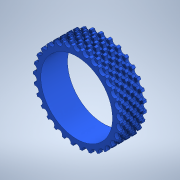
# Autodesk Inventor part: 3inBlueTread
Saved by Autodesk Inventor 2020 (Build 240168000, 168)
## iProperties
Created: 2019-05-28
Part Number: 3inBlueTread
Material: Generic
Document SubType Name: Modeling
Designer: Connor
Density: 1 g/cm^3
Appearance: Rubber - Blue
Author: Connor
Autodesk Inventor part; units mm, degrees
ref_plane "YZ Plane" through (0, 0, 0) normal (1, 0, 0) x (0, 1, 0)
ref_plane "XZ Plane" through (0, 0, 0) normal (0, 1, 0) x (-1, 0, 0)
ref_plane "XY Plane" through (0, 0, 0) normal (0, 0, 1) x (1, 0, 0)
sketch "Sketch1" plane through (0, 0, 0) normal (0, 0, 1) x (1, 0, 0)
  circle A0 centre (0, 0) radius 41.2242
  circle A1 centre (0, 0) radius 34.1122
  dimension "d3" = 7.112
  dimension "d4" = 68.2244
  constraints: 2 centre point, 1 coincident
  measures "d3" radial gap between concentric circles of A0 A1
  measures "d4" diameter of A1
extrude "Extrusion1" add sketch "Sketch1" along normal blind 25.4
sketch "Sketch3" plane through (0, 0, 25.4) normal (0, 0, 1) x (1, 0, 0)
  circle A0 centre (0, 0) radius 41.2242 projected
  arc A1 (-3.1726, 41.1019) -> (3.1726, 41.1019) centre (0, 41.2242) ccw
  circle A2 centre (0, 0) radius 41.2242 projected
  point P0 (-3.1726, 41.1019)
  point P1 (3.1726, 41.1019)
  dimension "d5" = 3.175
  constraints: 4 point on circle, 1 centre point, 1 vertical alignment, 2 other
  measures "d5" radius of A1
extrude "Extrusion2" cut sketch "Sketch3" against normal blind 3.175 contours A1 A0 picked at (0.1245, 40.1642)
pattern_circular "Circular Pattern3" count 30 over 360 about axis through (0, 0, 0) along (0, 0, 1) of "Extrusion2"
sketch "Sketch5" plane through (0, 0, 22.225) normal (0, 0, 1) x (1, 0, 0)
  arc A0 (-3.1726, 41.1019) -> (-5.4423, 40.8634) centre (0, 0) ccw projected
  circle A1 centre (0, 0) radius 41.2242 projected
  arc A2 (0.2324, 41.2235) -> (6.556, 40.6996) centre (3.4043, 41.0834) ccw
  arc A3 (3.1726, 41.1019) -> (-3.1726, 41.1019) centre (0, 0) ccw projected
  point P0 (3.6358, 41.0636)
  point P1 (0.2324, 41.2235)
  dimension "d30" = 3.175
  constraints: 6 point on circle, 1 centre point
  measures "d30" radius of A2
extrude "Extrusion4" cut sketch "Sketch5" against normal blind 3.175 contours A1 A2
pattern_circular "Circular Pattern4" count 30 over 360 about axis through (0, 0, 0) along (0, 0, 1) of "Extrusion4"
pattern_linear "Rectangular Pattern2" count 4 spacing 6.35 along (0, 0, -1) of "Extrusion4", "Circular Pattern4", "Extrusion2", "Circular Pattern3"
body "Solid1"
